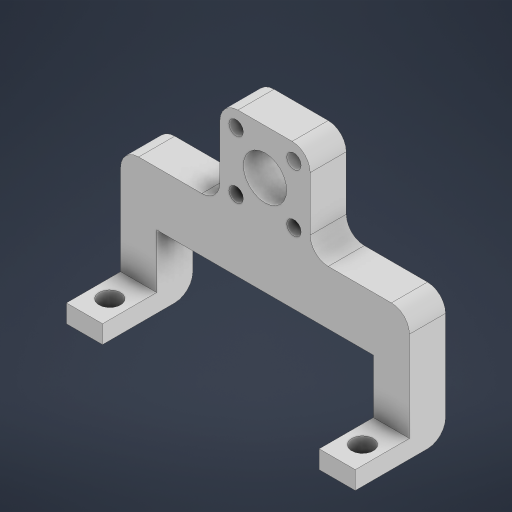
# Autodesk Inventor part: Bracket vorne
Saved by Autodesk Inventor 2023.2 (Build 272271000, 271)
## iProperties
Created: 2023-04-14
Part Number: Bracket vorne
Material: Generisch
Document SubType Name: Modeling
Designer: tadeus
Density: 1 g/cm^3
Appearance: Vorgabe
Author: tadeus
Autodesk Inventor part; units mm, degrees
ref_plane "YZ Plane" through (0, 0, 0) normal (1, 0, 0) x (0, 1, 0)
ref_plane "XZ Plane" through (0, 0, 0) normal (0, 1, 0) x (-1, 0, 0)
ref_plane "XY Plane" through (0, 0, 0) normal (0, 0, 1) x (1, 0, 0)
sketch "Skizze1" plane through (0, 0, 0) normal (0, 1, 0) x (-1, 0, 0)
  line L0 (40, -5) -> (-40, -5)
  line L1 (-40, -5) -> (-40, 5)
  line L2 (-40, 5) -> (-30, 5)
  line L3 (40, 5) -> (40, -5)
  line L4 (40, -5) -> (-40, 5) construction
  line L5 (-40, -5) -> (40, 5) construction
  line L6 (40, 5) -> (30, 5)
  line L7 (30, 5) -> (30, 20)
  line L8 (30, 20) -> (40, 20)
  line L9 (40, 20) -> (40, 5)
  circle A0 centre (35, 13) radius 3
  line L10 (0, 43.2114) -> (0, -35.1785) construction
  line L11 (-30, 5) -> (-30, 20)
  line L12 (-30, 20) -> (-40, 20)
  line L13 (-40, 20) -> (-40, 5)
  circle A1 centre (-35, 13) radius 3
  line L14 (-30, 5) -> (30, 5)
  line L15 (30, 5) -> (40, 5)
  line L16 (30, 5) -> (30, -5)
  line L17 (-30, 5) -> (-30, -5)
  point P0 (0, 0)
  point P1 (30, 12.5)
  dimension "d0" = 80
  dimension "d1" = 10
  dimension "d4" = 10
  dimension "d5" = 15
  dimension "d6" = 6
  dimension "d7" = 7
  dimension "d8" = 5
  constraints: 36 end point, 6 parallel, 4 symmetric about line, 3 midpoint, 3 perpendicular, 3 vertical, 2 centre point, 2 horizontal, 2 point on line, 1 other
  measures "d0" distance of L1.end L3.start
  measures "d1" distance of L0.end L1.end
  measures "d4" distance of L7.end L8.end
  measures "d5" distance of L6.end L7.end
  measures "d6" diameter of A0
  measures "d7" distance from line of L8 A0.centre
  measures "d8" horizontal distance of point (30, 12.5) A0.centre
extrude "Extrusion1" add sketch "Skizze1" along normal blind 60 contours L0 L16 L6 L3 | L0 L17 L14 L16 | L0 L1 L2 L17
extrude "Extrusion2" add sketch "Skizze1" along normal blind 5 contours L6 L7 L8 L9 | L2 L13 L12 L11
extrude "Extrusion3" cut sketch "Skizze1" along normal blind 20 contours L0 L17 L14 L16
sketch "Skizze2" plane through (-40, 60, 5) normal (0, 0, 1) x (1, 0, 0)
  line L0 (40, -60) -> (40, 40) construction
  circle A0 centre (32, -4.5) radius 2
  line L1 (70, -60) -> (80, -60) projected
  line L2 (40, -12.5) -> (0, -12.5) construction
  line L3 (0, -55) -> (0, 0) construction
  circle A1 centre (48, -4.5) radius 2
  circle A2 centre (32, -20.5) radius 2
  circle A3 centre (48, -20.5) radius 2
  circle A4 centre (40, -12.5) radius 6
  line L4 (0, 0) -> (80, 0) projected
  line L5 (27.5, -25) -> (52.5, -25)
  line L6 (52.5, -25) -> (52.5, 0)
  line L7 (52.5, 0) -> (27.5, 0)
  line L8 (27.5, 0) -> (27.5, -25)
  line L9 (27.5, -25) -> (52.5, 0) construction
  line L10 (52.5, -25) -> (27.5, 0) construction
  line L11 (27.5, -25) -> (0, -25)
  line L12 (0, -25) -> (0, 0)
  line L13 (0, 0) -> (27.5, 0)
  line L14 (27.5, 0) -> (27.5, -25)
  line L15 (80, -55) -> (80, 0) projected
  line L16 (52.5, -25) -> (80, -25)
  line L17 (80, -25) -> (80, 0)
  line L18 (80, 0) -> (52.5, 0)
  line L19 (52.5, 0) -> (52.5, -25)
  dimension "d14" = 4
  dimension "d15" = 47.5
  dimension "d16" = 8
  dimension "d17" = 8
  dimension "d20" = 16
  dimension "d23" = 16
  dimension "d26" = 12
  dimension "d27" = 25
  constraints: 32 end point, 6 parallel, 5 centre point, 5 horizontal, 3 perpendicular, 3 point on line, 2 midpoint, 2 vertical, 1 coincident, 6 other
  measures "d14" diameter of A0
  measures "d15" distance from line of L1 L2.start
  measures "d16" distance from line of L0 A0.centre
  measures "d17" distance from line of L2 A0.centre
  measures "d20" distance of A0.centre A1.centre
  measures "d23" distance of A0.centre A2.centre
  measures "d26" diameter of A4
  measures "d27" distance of L7.end L6.end
extrude "Extrusion4" cut sketch "Skizze2" against normal up to surface (10 mm away) contours A0 | A1 | A2 | A3 | A4 | L4 L8 L11 L12 | L4 L15 L16 L6
fillet "Rundung1" radius 5 8 edges at (-40, 35, 0) (-12.5, 35, 0) (-12.5, 60, 0) (12.5, 60, 0) (12.5, 35, 0) (40, 35, 0) (-35, 0, -5) (35, 0, -5)
